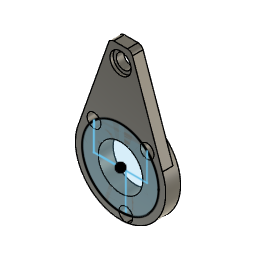
support volant keya claas (v1~recovered) (Autodesk Fusion 360 design; units mm, degrees)
Autodesk Fusion 360 part; units mm, degrees
note: some values were not read from the file. Set by a fixed rule: the direction of a hole.
sketch "Esquisse1" plane through (0, 0, 0) normal (0, 1, 0) x (1, 0, 0)
  circle A0 centre (0, 0) radius 42.5
  circle A1 centre (0, 0) radius 21
  line L0 (0, 0) -> (0, -100)
  line L1 (0, -100) -> (-10, -100)
  line L2 (0, -100) -> (10, -100)
  line L3 (-10, -100) -> (-39.346862, -16.064695)
  line L4 (10, -100) -> (39.346941, -16.064502)
  dimension "d1" = 85
  dimension "d2" = 42
  dimension "d3" = 100
  dimension "d4" = 10
  dimension "d5" = 10
  dimension "d6" = 88.918
  constraint coincident A0.centre A1.centre
  constraint vertical L0
  constraint perpendicular L0 L1
  constraint perpendicular L0 L2
  measures "d1" diameter of A0
  measures "d2" diameter of A1
  measures "d3" distance of A0.centre L0.end
  measures "d4" distance of L0.end L1.end
  measures "d5" distance of L0.end L2.end
extrude "Extrusion1" add sketch "Esquisse1" along normal blind 10 contours A0 L0 L1 L3 | A0 L0 L2 L4 picked at (-3.333333, -80.833333) picked at (3.333333, -80.833333)
extrude "Extrusion2" add sketch "Esquisse1" along normal blind 14 contours A0 picked at (31.666459, -15.491813)
fillet "Congé1" radius 5 1 edges at (10, 5, 100)
fillet "Congé2" radius 5 1 edges at (-10, 5, 100)
sketch "Esquisse2" plane through (0, 0, 0) normal (0, 1, 0) x (1, 0, 0)
  circle A0 centre (0, 0) radius 36
  line L0 (0, 0) -> (25, 0)
  line L1 (0, 0) -> (-25, 0)
  line L2 (-25, 0) -> (-25, -25.903668)
  line L3 (25, 0) -> (25, -25.903668)
  dimension "d15" = 72
  dimension "d16" = 25
  dimension "d17" = 25
  constraint coincident A0.centre L0.start
  constraint perpendicular L1 L2
  constraint perpendicular L0 L3
  measures "d15" diameter of A0
  measures "d16" distance of A0.centre L0.end
  measures "d17" distance of A0.centre L1.end
hole "Perçage1" at (25, 0, 25.903668) direction (0, 1, 0) diameter 7.5 depth 15 tip angle 180 counterbore diameter 13 counterbore depth 10
sketch "Esquisse3" plane through (0, 0, 0) normal (0, 1, 0) x (1, 0, 0)
  circle A0 centre (0, 0) radius 36
  line L0 (0, 0) -> (-25, 0)
  line L1 (-25, 0) -> (-25, -25.903668)
  dimension "d23" = 72
  dimension "d24" = 25
  constraint coincident A0.centre L0.start
  constraint perpendicular L0 L1
  measures "d23" diameter of A0
  measures "d24" distance of A0.centre L0.end
hole "Perçage2" at (-25, 0, 25.903668) direction (0, 1, 0) diameter 7.5 depth 15 tip angle 180 counterbore diameter 13 counterbore depth 10
sketch "Esquisse4" plane through (0, 0, 0) normal (0, 1, 0) x (1, 0, 0)
  circle A0 centre (0, 0) radius 36
  line L0 (0, 0) -> (5, 0)
  line L1 (5, 0) -> (5, 35.651087)
  dimension "d30" = 72
  dimension "d31" = 5
  constraint coincident A0.centre L0.start
  constraint perpendicular L0 L1
  measures "d30" diameter of A0
  measures "d31" distance of A0.centre L0.end
hole "Perçage3" at (5, 0, -35.651087) direction (0, 1, 0) diameter 7.5 depth 15 tip angle 180 counterbore diameter 13 counterbore depth 10
sketch "Esquisse5" plane through (0, 0, 0) normal (0, 1, 0) x (1, 0, 0)
  line L0 (0, 0) -> (0, -85)
  dimension "d37" = 85
  constraint coincident L0.start origin
  measures "d37" distance of L0.start L0.end
hole "Perçage4" at (0, 0, 85) direction (0, 1, 0) diameter 14 depth 10 tip angle 180 counterbore diameter 20 counterbore depth 3
